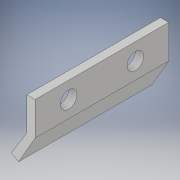
# Autodesk Inventor part: 2AM-17-P-5203 - flaps
Saved by Autodesk Inventor 2017 (Build 210142000, 142)
## iProperties
Created: 2017-12-28
Part Number: 2AM-17-P-5203 - flaps
Material: Generic
Document SubType Name: Modeling
Designer: Micah
Density: 1 g/cm^3
Appearance: Default
Author: Micah
Autodesk Inventor part; units mm, degrees
ref_plane "YZ Plane" through (0, 0, 0) normal (1, 0, 0) x (0, 1, 0)
ref_plane "XZ Plane" through (0, 0, 0) normal (0, 1, 0) x (-1, 0, 0)
ref_plane "XY Plane" through (0, 0, 0) normal (0, 0, 1) x (1, 0, 0)
sketch "Sketch2" plane through (0, 0, 0) normal (0, 0, 1) x (1, 0, 0)
  line L0 (0, 0) -> (-3.175, -5.4993)
  line L1 (0, 0) -> (6.35, 0) construction
  line L2 (0, 0) -> (0, 6.35)
  line L3 (0, 6.35) -> (-1.5875, 6.35)
  line L4 (-1.5875, 6.35) -> (-1.5875, 0)
  line L5 (-3.175, -5.4993) -> (-4.5498, -4.7055)
  line L6 (-4.5498, -4.7055) -> (-1.5875, 0)
  dimension "d0" = 6.35
  dimension "d1" = 120
  dimension "d2" = 6.35
  dimension "d3" = 1.5875
  dimension "d4" = 1.5875
  constraints: 14 end point, 2 vertical, 1 equal length, 1 horizontal, 1 perpendicular
  measures "d0" distance of L0.start L0.end
  measures "d1" angle of L0 L1
  measures "d2" distance of L0.start L2.end
  measures "d3" distance of L2.end L3.end
  measures "d4" distance of L0.end L5.end
extrude "Extrusion1" add sketch "Sketch2" along normal blind 25.4
sketch "Sketch3" plane through (-1.5875, 0, 0) normal (-1, 0, 0) x (0, 0, 1)
  line L0 (0, 6.35) -> (25.4, 6.35) projected
  line L1 (6.35, 6.35) -> (6.35, 0)
  line L2 (0, 0) -> (0, 6.35) projected
  line L3 (12.7, 6.35) -> (12.7, 0)
  line L4 (0, 0) -> (25.4, 0) projected
  circle A0 centre (6.35, 3.175) radius 1.5875
  circle A1 centre (19.05, 3.175) radius 1.5875
  dimension "d7" = 6.35
  dimension "d8" = 3.175
  constraints: 4 end point, 3 midpoint, 2 centre point, 1 perpendicular, 1 point on line, 1 symmetric about line, 1 other
  measures "d7" distance between parallel lines of L2 L1
  measures "d8" diameter of A0
hole "Hole1" at (-1.5875, 3.175, 6.35) at (-1.5875, 3.175, 19.05) direction (1, 0, 0) diameter 3.175 depth 25.4 tip angle 118
body "Solid1"
